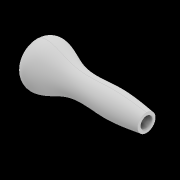
# Autodesk Inventor part: ShiftHandleV2
Saved by Autodesk Inventor 2022 (Build 260153000, 153)
## iProperties
Created: 2020-12-27
Part Number: ShiftHandleV2
Material: Generic
Document SubType Name: Modeling
Designer: jdski
Density: 1 g/cm^3
Appearance: Default
Author: jdski
Autodesk Inventor part; units mm, degrees
ref_plane "YZ Plane" through (0, 0, 0) normal (1, 0, 0) x (0, 1, 0)
ref_plane "XZ Plane" through (0, 0, 0) normal (0, 1, 0) x (-1, 0, 0)
ref_plane "XY Plane" through (0, 0, 0) normal (0, 0, 1) x (1, 0, 0)
sketch "Sketch2" plane through (0, 0, 0) normal (0, 0, 1) x (1, 0, 0)
  line L0 (29.7622, 3.0778) -> (-9.3535, 3.0778)
  spline S0 degree 3 poles (-15.3987, 4.6526) (-15.2053, 5.5483) (-14.8331, 7.2724) (-9.8973, 11.3764) (0.9526, 3.6094) (15.0147, 6.3749) (25.0703, 4.9293) (29.7622, 4.2547) knots 0 0 0 0 0.268945 0.517689 1.772192 3.385082 4.79595 4.79595 4.79595 4.79595
  line L1 (29.7622, 4.2547) -> (29.7622, 3.0778)
  line L2 (29.7622, 0.7156) -> (-24.086, 0.7156)
  line L3 (-15.3987, 4.6526) -> (-9.3535, 4.6526)
  line L4 (-15.3987, 4.6526) -> (-9.3535, 4.6526) construction
  line L5 (-9.3535, 4.6526) -> (-9.3535, 3.0778)
  point P0 (0, 0)
  point P1 (-14.5299, 7.1979)
  point P2 (-12.6698, 8.8493)
  point P3 (-0.4022, 6.2255)
  point P4 (15.712, 5.5381)
  dimension "d3" = 6.0452
  dimension "d5" = 1.5748
  constraints: 12 end point, 2 horizontal, 1 collinear, 6 other
  measures "d3" distance of L3.start L3.end
  measures "d5" distance of L3.end L0.end
revolve "Revolution2" add sketch "Sketch2" angle 360 about axis through (29.7622, 0.7156, 0) along (-1, 0, 0)
body "Solid2"
